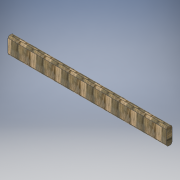
# Autodesk Inventor part: SideShort
Saved by Autodesk Inventor 2017 (Build 210142000, 142)
## iProperties
Created: 2016-10-24
Part Number: SideShort
Material: Generic
Document SubType Name: Modeling
Designer: andrew
Density: 1 g/cm^3
Appearance: Driftwood
d0: 33.000 in
Author: andrew
Autodesk Inventor part; units mm, degrees
ref_plane "YZ Plane" through (0, 0, 0) normal (1, 0, 0) x (0, 1, 0)
ref_plane "XZ Plane" through (0, 0, 0) normal (0, 1, 0) x (-1, 0, 0)
ref_plane "XY Plane" through (0, 0, 0) normal (0, 0, 1) x (1, 0, 0)
sketch "Sketch1" plane through (0, 0, 0) normal (0, 0, 1) x (1, 0, 0)
  line L0 (-419.1, -44.45) -> (419.1, -44.45)
  line L1 (419.1, -44.45) -> (419.1, 44.45)
  line L2 (419.1, 44.45) -> (-419.1, 44.45)
  line L3 (-419.1, 44.45) -> (-419.1, -44.45)
  line L4 (-419.1, -44.45) -> (419.1, 44.45) construction
  line L5 (419.1, -44.45) -> (-419.1, 44.45) construction
  point P0 (0, 0)
  dimension "d0" = 838.2
  dimension "d1" = 88.9
  constraints: 12 end point, 2 midpoint, 2 parallel, 1 horizontal, 1 perpendicular
  measures "d0" distance of L1.end L2.end
  measures "d1" distance of L2.end L0.start
extrude "Extrusion1" add sketch "Sketch1" along normal blind 28.575
fillet "Fillet1" radius 9.525 4 edges at (0, 44.45, 28.575) (0, 44.45, 0) (0, -44.45, 0) (0, -44.45, 28.575)
body "Solid1"
